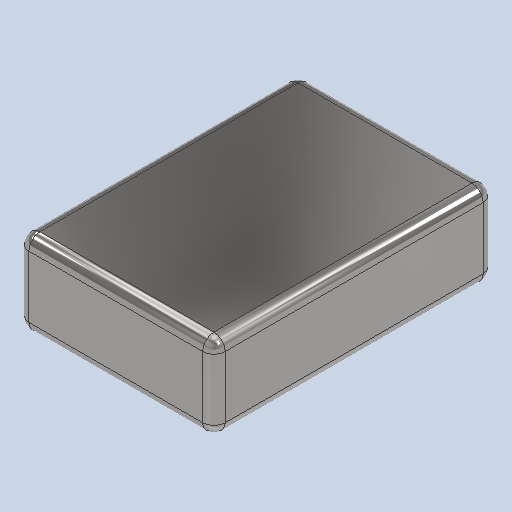
# Autodesk Inventor part: stator_magnet
Saved by Autodesk Inventor 2025 (Build 290162000, 162)
## iProperties
Created: 2026-08-03
Part Number: stator_magnet
Material: Ogólny
Document SubType Name: Modeling
Designer: zzapa
Density: 1 g/cm^3
Appearance: Stal — polerowana
Mass: 0.207339 g
Surface Area: 2.28084 cm^2
Volume: 0.207339 cm^3
Author: zzapa
Autodesk Inventor part; units mm, degrees
ref_plane "YZ Plane" through (0, 0, 0) normal (1, 0, 0) x (0, 1, 0)
ref_plane "XZ Plane" through (0, 0, 0) normal (0, 1, 0) x (-1, 0, 0)
ref_plane "XY Plane" through (0, 0, 0) normal (0, 0, 1) x (1, 0, 0)
sketch "Szkic1" plane through (0, 0, 0) normal (0, 1, 0) x (-1, 0, 0)
  line L0 (3.5, 5) -> (-3.5, 5)
  line L1 (-3.5, 5) -> (-3.5, -5)
  line L2 (-3.5, -5) -> (3.5, -5)
  line L3 (3.5, -5) -> (3.5, 5)
  line L4 (4.9, 0) -> (-4.9, 0) projected
  line L5 (0, -7) -> (0, 7) projected
  point P0 (0, 0)
  point P1 (3.5, 0)
  point P2 (0, 5)
  dimension "d0" = 7
  dimension "d1" = 10
  constraints: 8 end point, 2 midpoint, 2 parallel, 2 point on line, 1 horizontal, 1 perpendicular
  measures "d0" distance of L1.end L2.end
  measures "d1" distance of L2.end L0.start
extrude "Wyciągnięcie proste1" add sketch "Szkic1" along normal blind 3
fillet "Zaokrąglenie1" radius 0.4 12 edges at (0, 3, 5) (3.5, 3, 0) (0, 0, 5) (3.5, 0, 0) (3.5, 1.5, 5) (3.5, 1.5, -5) (0, 3, -5) (0, 0, -5) (-3.5, 1.5, -5) (-3.5, 3, 0) (-3.5, 0, 0) (-3.5, 1.5, 5)
equation "\"d0\" = mag_size_x"
equation "\"d1\" = mag_size_z"
equation "\"d2\" = mag_size_y"
equation "\"d4\" = mag_corner_r"
equation "\"stator_out_d\" = 2.5"
equation "\"stator_h\" = 35"
equation "\"mag_size_x\" = 7"
equation "\"mag_size_y\" = 3"
equation "\"mag_size_z\" = 10"
equation "\"mag_corner_r\" = 0.4"
equation "\"magnet_ring_d\" = 3.3"
equation "\"magnet_ring_r\" = 27.5"
equation "\"magnet_ring_pocket_mag_size_y\" = 3.1"
equation "\"magnet_ring_pocket_mag_size_x\" = 7.1"
equation "\"magnet_ring_pocket_mag_size_z\" = 10.3"
equation "\"magnet_ring_mag_count\" = 16"
equation "\"magnet_ring_h\" = 36"
equation "\"magnet_ring_pocket_radial_cut\" = 1.4"
equation "\"casing_d\" = 3"
equation "\"rotor_core_r\" = 15"
equation "\"coil_groove_ang\" = 18"
equation "\"rotor_out_r\" = 23"
equation "\"rotor_coil_groove_in_r\" = 17"
equation "\"rotor_coil_groove_ang\" = 18deg"
equation "\"rotor_coil_groove_in_correction_r\" = 18"
equation "\"rotor_plastic_h\" = 32"
equation "\"rotor_teeth_d\" = 1.5"
equation "\"shaft_d\" = 8"
equation "\"insert25m_d\" = 2.9"
equation "\"insert25m_corner\" = 0.5"
equation "\"insert25m_h\" = 7"
equation "\"rotor_plastic_insert_r\" = 37"
equation "\"shaft_lock_1_d\" = 8"
equation "\"shaf_lock_1_D\" = 32"
equation "\"shaft_lock_1_D\" = 36"
equation "\"shaft_lock_1_h1\" = 4"
equation "\"shaft_lock_1_insert_part_h\" = 7"
equation "\"shaft_lock_1_corner\" = 1"
equation "\"shaft_lock_1_insert_part_a\" = 18"
equation "\"shaft_lock_2_h1\" = 4"
equation "\"shaft_lock_2_d\" = 7"
equation "\"shaft_lock_2_insert_part_a\" = 18"
equation "\"shaft_lock_2_D\" = 44"
equation "\"shaft_lock_2_corner\" = 1"
equation "\"shaft_lock_2_insert_part_h\" = 7"
equation "\"shaft_lock_2_rotor_insert_grove_d_in\" = 36"
equation "\"shaft_lock_2_rotor_insert_grove_width_out\" = 5.5"
equation "\"shaft_lock_2_rotor_insert_grove_width_in\" = 7.6"
equation "\"shaft_lock_2_rotor_insert_r\" = 37"
equation "\"shaft_lock_2_rotor_insert_screw_d\" = 2.6"
equation "\"insert25m_pocket_d\" = 2.6"
equation "\"insert25m_pocket_D\" = 4.5"
equation "\"insert25m_pocket_nut_h\" = 1.5"
equation "\"insert_m2_pocket_d\" = 2.6"
equation "\"insert_m2_h\" = 7"
equation "\"insert_m2_d\" = 2.9"
equation "\"insert_m2_corner\" = 0.5"
equation "\"insert_m2_pocket_D\" = 4.5"
equation "\"insert_m2_pocket_nut_h\" = 1.5"
